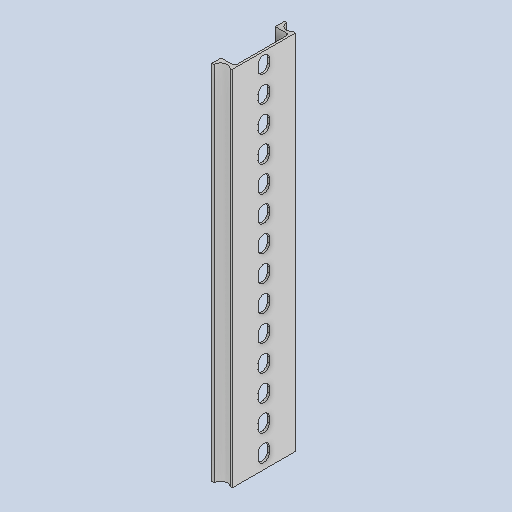
# Autodesk Inventor part: CB_dinrail_mk
Saved by Autodesk Inventor 2022 (Build 260153070, 153G)
## iProperties
Created: 2022-06-25
Part Number: CB_dinrail_mk
Material: アルミニウム 6061-AHC
Document SubType Name: Modeling
Designer: sky
Density: 2.7 g/cm^3
Appearance: アルミニウム - ダーク
Author: sky
Autodesk Inventor part; units mm, degrees
ref_plane "YZ Plane" through (0, 0, 0) normal (1, 0, 0) x (0, 1, 0)
ref_plane "XZ Plane" through (0, 0, 0) normal (0, 1, 0) x (-1, 0, 0)
ref_plane "XY Plane" through (0, 0, 0) normal (0, 0, 1) x (1, 0, 0)
sketch "スケッチ1" plane through (0, 0, 0) normal (0, 1, 0) x (-1, 0, 0)
  line L0 (0, 0) -> (0, -30.5)
  line L1 (7.5, 2.25) -> (7.5, -32.75)
  line L2 (11.9991, -15.25) -> (-11.598, -15.25)
  line L3 (7.5, 2.25) -> (6.5, 2.25)
  line L4 (7.5, 2.25) -> (8.5, 2.25) construction
  line L5 (0, 0) -> (1, 0)
  arc A0 (1, 0) -> (6.5, 2.25) centre (3.2952, 2.2367) ccw
  line L6 (7.5, -32.75) -> (6.5, -32.75)
  line L7 (0, -30.5) -> (1, -30.5)
  arc A1 (6.5, -32.75) -> (1, -30.5) centre (3.2952, -32.7367) ccw
  line L8 (7.5, -2.15) -> (1, -2.15)
  line L9 (1, -2.15) -> (1, -28.35)
  line L10 (1, -28.35) -> (7.5, -28.35)
  dimension "d0" = 30.5
  dimension "d1" = 35
  dimension "d2" = 7.5
  dimension "d3" = 2.25
  dimension "d4" = 1
  dimension "d5" = 180
  dimension "d6" = 1
  dimension "d7" = 4.4
  dimension "d8" = 4.4
  constraints: 22 end point, 5 horizontal, 4 point on circle, 3 symmetric about line, 2 centre point, 2 point on line, 2 vertical, 1 collinear, 1 parallel, 1 perpendicular, 1 other
  measures "d0" distance of L0.start L0.end
  measures "d1" distance of L1.start L1.end
  measures "d2" distance between parallel lines of L1 L0
  measures "d3" vertical distance of L0.start L1.start
  measures "d4" distance of L1.start L3.end
  measures "d5" angle of L3 L4
  measures "d6" distance of L0.start L5.end
  measures "d7" distance between parallel lines of L8 L3
  measures "d8" distance between parallel lines of L10 L6
extrude "押し出し1" add sketch "スケッチ1" along normal blind 175 contours L5 A0 L3 L1 L8 L9 L2 L0 | L2 L9 L10 L1 L6 A1 L7 L0
sketch "スケッチ2" plane through (-1, 0, -28.35) normal (-1, 0, 0) x (0, 0, 1)
  line L0 (0, 0) -> (26.2, 0) projected
  line L1 (26.2, 0) -> (26.2, 175) projected
  line L2 (0, 175) -> (26.2, 175) projected
  line L3 (0, 0) -> (0, 175) projected
  line L4 (15.85, 3) -> (10.35, 3)
  line L5 (10.35, 3) -> (10.35, 11)
  line L6 (10.35, 11) -> (15.85, 11)
  line L7 (15.85, 11) -> (15.85, 3)
  arc A0 (13.1, 3) -> (15.85, 5.75) centre (13.1, 5.75) ccw
  arc A1 (10.35, 5.75) -> (13.1, 3) centre (13.1, 5.75) ccw
  arc A2 (13.1, 11) -> (10.35, 8.25) centre (13.1, 8.25) ccw
  arc A3 (15.85, 8.25) -> (13.1, 11) centre (13.1, 8.25) ccw
  line L8 (15.85, 15.5) -> (10.35, 15.5)
  arc A4 (13.1, 15.5) -> (15.85, 18.25) centre (13.1, 18.25) ccw
  arc A5 (10.35, 18.25) -> (13.1, 15.5) centre (13.1, 18.25) ccw
  arc A6 (15.85, 20.75) -> (13.1, 23.5) centre (13.1, 20.75) ccw
  arc A7 (13.1, 23.5) -> (10.35, 20.75) centre (13.1, 20.75) ccw
  line L9 (10.35, 15.5) -> (10.35, 23.5)
  line L10 (15.85, 23.5) -> (15.85, 15.5)
  line L11 (15.85, 28) -> (10.35, 28)
  arc A8 (13.1, 28) -> (15.85, 30.75) centre (13.1, 30.75) ccw
  arc A9 (10.35, 30.75) -> (13.1, 28) centre (13.1, 30.75) ccw
  arc A10 (15.85, 33.25) -> (13.1, 36) centre (13.1, 33.25) ccw
  arc A11 (13.1, 36) -> (10.35, 33.25) centre (13.1, 33.25) ccw
  line L12 (10.35, 28) -> (10.35, 36)
  line L13 (15.85, 36) -> (15.85, 28)
  line L14 (15.85, 40.5) -> (10.35, 40.5)
  arc A12 (13.1, 40.5) -> (15.85, 43.25) centre (13.1, 43.25) ccw
  arc A13 (10.35, 43.25) -> (13.1, 40.5) centre (13.1, 43.25) ccw
  arc A14 (15.85, 45.75) -> (13.1, 48.5) centre (13.1, 45.75) ccw
  arc A15 (13.1, 48.5) -> (10.35, 45.75) centre (13.1, 45.75) ccw
  line L15 (10.35, 40.5) -> (10.35, 48.5)
  line L16 (15.85, 48.5) -> (15.85, 40.5)
  line L17 (15.85, 53) -> (10.35, 53)
  arc A16 (13.1, 53) -> (15.85, 55.75) centre (13.1, 55.75) ccw
  arc A17 (10.35, 55.75) -> (13.1, 53) centre (13.1, 55.75) ccw
  arc A18 (15.85, 58.25) -> (13.1, 61) centre (13.1, 58.25) ccw
  arc A19 (13.1, 61) -> (10.35, 58.25) centre (13.1, 58.25) ccw
  line L18 (10.35, 53) -> (10.35, 61)
  line L19 (15.85, 61) -> (15.85, 53)
  line L20 (15.85, 65.5) -> (10.35, 65.5)
  arc A20 (13.1, 65.5) -> (15.85, 68.25) centre (13.1, 68.25) ccw
  arc A21 (10.35, 68.25) -> (13.1, 65.5) centre (13.1, 68.25) ccw
  arc A22 (15.85, 70.75) -> (13.1, 73.5) centre (13.1, 70.75) ccw
  arc A23 (13.1, 73.5) -> (10.35, 70.75) centre (13.1, 70.75) ccw
  line L21 (10.35, 65.5) -> (10.35, 73.5)
  line L22 (15.85, 73.5) -> (15.85, 65.5)
  line L23 (15.85, 78) -> (10.35, 78)
  arc A24 (13.1, 78) -> (15.85, 80.75) centre (13.1, 80.75) ccw
  arc A25 (10.35, 80.75) -> (13.1, 78) centre (13.1, 80.75) ccw
  arc A26 (15.85, 83.25) -> (13.1, 86) centre (13.1, 83.25) ccw
  arc A27 (13.1, 86) -> (10.35, 83.25) centre (13.1, 83.25) ccw
  line L24 (10.35, 78) -> (10.35, 86)
  line L25 (15.85, 86) -> (15.85, 78)
  line L26 (15.85, 90.5) -> (10.35, 90.5)
  arc A28 (13.1, 90.5) -> (15.85, 93.25) centre (13.1, 93.25) ccw
  arc A29 (10.35, 93.25) -> (13.1, 90.5) centre (13.1, 93.25) ccw
  arc A30 (15.85, 95.75) -> (13.1, 98.5) centre (13.1, 95.75) ccw
  arc A31 (13.1, 98.5) -> (10.35, 95.75) centre (13.1, 95.75) ccw
  line L27 (10.35, 90.5) -> (10.35, 98.5)
  line L28 (15.85, 98.5) -> (15.85, 90.5)
  line L29 (15.85, 103) -> (10.35, 103)
  arc A32 (13.1, 103) -> (15.85, 105.75) centre (13.1, 105.75) ccw
  arc A33 (10.35, 105.75) -> (13.1, 103) centre (13.1, 105.75) ccw
  arc A34 (15.85, 108.25) -> (13.1, 111) centre (13.1, 108.25) ccw
  arc A35 (13.1, 111) -> (10.35, 108.25) centre (13.1, 108.25) ccw
  line L30 (10.35, 103) -> (10.35, 111)
  line L31 (15.85, 111) -> (15.85, 103)
  line L32 (15.85, 115.5) -> (10.35, 115.5)
  arc A36 (13.1, 115.5) -> (15.85, 118.25) centre (13.1, 118.25) ccw
  arc A37 (10.35, 118.25) -> (13.1, 115.5) centre (13.1, 118.25) ccw
  arc A38 (15.85, 120.75) -> (13.1, 123.5) centre (13.1, 120.75) ccw
  arc A39 (13.1, 123.5) -> (10.35, 120.75) centre (13.1, 120.75) ccw
  line L33 (10.35, 115.5) -> (10.35, 123.5)
  line L34 (15.85, 123.5) -> (15.85, 115.5)
  line L35 (15.85, 128) -> (10.35, 128)
  arc A40 (13.1, 128) -> (15.85, 130.75) centre (13.1, 130.75) ccw
  arc A41 (10.35, 130.75) -> (13.1, 128) centre (13.1, 130.75) ccw
  arc A42 (15.85, 133.25) -> (13.1, 136) centre (13.1, 133.25) ccw
  arc A43 (13.1, 136) -> (10.35, 133.25) centre (13.1, 133.25) ccw
  line L36 (10.35, 128) -> (10.35, 136)
  line L37 (15.85, 136) -> (15.85, 128)
  line L38 (15.85, 140.5) -> (10.35, 140.5)
  arc A44 (13.1, 140.5) -> (15.85, 143.25) centre (13.1, 143.25) ccw
  arc A45 (10.35, 143.25) -> (13.1, 140.5) centre (13.1, 143.25) ccw
  arc A46 (15.85, 145.75) -> (13.1, 148.5) centre (13.1, 145.75) ccw
  arc A47 (13.1, 148.5) -> (10.35, 145.75) centre (13.1, 145.75) ccw
  line L39 (10.35, 140.5) -> (10.35, 148.5)
  line L40 (15.85, 148.5) -> (15.85, 140.5)
  line L41 (15.85, 153) -> (10.35, 153)
  arc A48 (13.1, 153) -> (15.85, 155.75) centre (13.1, 155.75) ccw
  arc A49 (10.35, 155.75) -> (13.1, 153) centre (13.1, 155.75) ccw
  arc A50 (15.85, 158.25) -> (13.1, 161) centre (13.1, 158.25) ccw
  arc A51 (13.1, 161) -> (10.35, 158.25) centre (13.1, 158.25) ccw
  line L42 (10.35, 153) -> (10.35, 161)
  line L43 (15.85, 161) -> (15.85, 153)
  line L44 (15.85, 165.5) -> (10.35, 165.5)
  arc A52 (13.1, 165.5) -> (15.85, 168.25) centre (13.1, 168.25) ccw
  arc A53 (10.35, 168.25) -> (13.1, 165.5) centre (13.1, 168.25) ccw
  arc A54 (15.85, 170.75) -> (13.1, 173.5) centre (13.1, 170.75) ccw
  arc A55 (13.1, 173.5) -> (10.35, 170.75) centre (13.1, 170.75) ccw
  line L45 (10.35, 165.5) -> (10.35, 173.5)
  line L46 (15.85, 173.5) -> (15.85, 165.5)
  line L47 (15.85, 178) -> (10.35, 178)
  arc A56 (13.1, 178) -> (15.85, 180.75) centre (13.1, 180.75) ccw
  arc A57 (10.35, 180.75) -> (13.1, 178) centre (13.1, 180.75) ccw
  arc A58 (15.85, 183.25) -> (13.1, 186) centre (13.1, 183.25) ccw
  arc A59 (13.1, 186) -> (10.35, 183.25) centre (13.1, 183.25) ccw
  line L48 (10.35, 178) -> (10.35, 186)
  line L49 (15.85, 186) -> (15.85, 178)
  line L50 (15.85, 190.5) -> (10.35, 190.5)
  arc A60 (13.1, 190.5) -> (15.85, 193.25) centre (13.1, 193.25) ccw
  arc A61 (10.35, 193.25) -> (13.1, 190.5) centre (13.1, 193.25) ccw
  arc A62 (15.85, 195.75) -> (13.1, 198.5) centre (13.1, 195.75) ccw
  arc A63 (13.1, 198.5) -> (10.35, 195.75) centre (13.1, 195.75) ccw
  line L51 (10.35, 190.5) -> (10.35, 198.5)
  line L52 (15.85, 198.5) -> (15.85, 190.5)
  line L53 (15.85, 203) -> (10.35, 203)
  arc A64 (13.1, 203) -> (15.85, 205.75) centre (13.1, 205.75) ccw
  arc A65 (10.35, 205.75) -> (13.1, 203) centre (13.1, 205.75) ccw
  arc A66 (15.85, 208.25) -> (13.1, 211) centre (13.1, 208.25) ccw
  arc A67 (13.1, 211) -> (10.35, 208.25) centre (13.1, 208.25) ccw
  line L54 (10.35, 203) -> (10.35, 211)
  line L55 (15.85, 211) -> (15.85, 203)
  line L56 (15.85, 215.5) -> (10.35, 215.5)
  arc A68 (13.1, 215.5) -> (15.85, 218.25) centre (13.1, 218.25) ccw
  arc A69 (10.35, 218.25) -> (13.1, 215.5) centre (13.1, 218.25) ccw
  arc A70 (15.85, 220.75) -> (13.1, 223.5) centre (13.1, 220.75) ccw
  arc A71 (13.1, 223.5) -> (10.35, 220.75) centre (13.1, 220.75) ccw
  line L57 (10.35, 215.5) -> (10.35, 223.5)
  line L58 (15.85, 223.5) -> (15.85, 215.5)
  line L59 (15.85, 228) -> (10.35, 228)
  arc A72 (13.1, 228) -> (15.85, 230.75) centre (13.1, 230.75) ccw
  arc A73 (10.35, 230.75) -> (13.1, 228) centre (13.1, 230.75) ccw
  arc A74 (15.85, 233.25) -> (13.1, 236) centre (13.1, 233.25) ccw
  arc A75 (13.1, 236) -> (10.35, 233.25) centre (13.1, 233.25) ccw
  line L60 (10.35, 228) -> (10.35, 236)
  line L61 (15.85, 236) -> (15.85, 228)
  line L62 (15.85, 240.5) -> (10.35, 240.5)
  arc A76 (13.1, 240.5) -> (15.85, 243.25) centre (13.1, 243.25) ccw
  arc A77 (10.35, 243.25) -> (13.1, 240.5) centre (13.1, 243.25) ccw
  arc A78 (15.85, 245.75) -> (13.1, 248.5) centre (13.1, 245.75) ccw
  arc A79 (13.1, 248.5) -> (10.35, 245.75) centre (13.1, 245.75) ccw
  line L63 (10.35, 240.5) -> (10.35, 248.5)
  line L64 (15.85, 248.5) -> (15.85, 240.5)
  line L65 (15.85, 253) -> (10.35, 253)
  arc A80 (13.1, 253) -> (15.85, 255.75) centre (13.1, 255.75) ccw
  arc A81 (10.35, 255.75) -> (13.1, 253) centre (13.1, 255.75) ccw
  arc A82 (15.85, 258.25) -> (13.1, 261) centre (13.1, 258.25) ccw
  arc A83 (13.1, 261) -> (10.35, 258.25) centre (13.1, 258.25) ccw
  line L66 (10.35, 253) -> (10.35, 261)
  line L67 (15.85, 261) -> (15.85, 253)
  line L68 (15.85, 265.5) -> (10.35, 265.5)
  arc A84 (13.1, 265.5) -> (15.85, 268.25) centre (13.1, 268.25) ccw
  arc A85 (10.35, 268.25) -> (13.1, 265.5) centre (13.1, 268.25) ccw
  arc A86 (15.85, 270.75) -> (13.1, 273.5) centre (13.1, 270.75) ccw
  arc A87 (13.1, 273.5) -> (10.35, 270.75) centre (13.1, 270.75) ccw
  line L69 (10.35, 265.5) -> (10.35, 273.5)
  line L70 (15.85, 273.5) -> (15.85, 265.5)
  line L71 (15.85, 278) -> (10.35, 278)
  arc A88 (13.1, 278) -> (15.85, 280.75) centre (13.1, 280.75) ccw
  arc A89 (10.35, 280.75) -> (13.1, 278) centre (13.1, 280.75) ccw
  arc A90 (15.85, 283.25) -> (13.1, 286) centre (13.1, 283.25) ccw
  arc A91 (13.1, 286) -> (10.35, 283.25) centre (13.1, 283.25) ccw
  line L72 (10.35, 278) -> (10.35, 286)
  line L73 (15.85, 286) -> (15.85, 278)
  line L74 (15.85, 290.5) -> (10.35, 290.5)
  arc A92 (13.1, 290.5) -> (15.85, 293.25) centre (13.1, 293.25) ccw
  arc A93 (10.35, 293.25) -> (13.1, 290.5) centre (13.1, 293.25) ccw
  arc A94 (15.85, 295.75) -> (13.1, 298.5) centre (13.1, 295.75) ccw
  arc A95 (13.1, 298.5) -> (10.35, 295.75) centre (13.1, 295.75) ccw
  line L75 (10.35, 290.5) -> (10.35, 298.5)
  line L76 (15.85, 298.5) -> (15.85, 290.5)
  line L77 (15.85, 303) -> (10.35, 303)
  arc A96 (13.1, 303) -> (15.85, 305.75) centre (13.1, 305.75) ccw
  arc A97 (10.35, 305.75) -> (13.1, 303) centre (13.1, 305.75) ccw
  arc A98 (15.85, 308.25) -> (13.1, 311) centre (13.1, 308.25) ccw
  arc A99 (13.1, 311) -> (10.35, 308.25) centre (13.1, 308.25) ccw
  line L78 (10.35, 303) -> (10.35, 311)
  line L79 (15.85, 311) -> (15.85, 303)
  point P0 (28.35, 0)
  dimension "d11" = 5.5
  dimension "d12" = 8
  dimension "d13" = 10.35
  dimension "d14" = 3
  dimension "d16" = 2.75
  dimension "d18" = 2.75
  dimension "d21" = 12.5
  constraints: 200 point on circle, 152 end point, 100 centre point, 100 point on line, 26 midpoint, 2 parallel, 1 collinear, 1 horizontal, 1 perpendicular, 1 vertical, 455 other
  measures "d11" distance of L5.end L6.end
  measures "d12" distance of L4.end L5.end
  measures "d13" distance between parallel lines of L3 L5
  measures "d14" distance between parallel lines of L0 L4
  measures "d16" distance from line of L6 A2.centre
  measures "d18" distance from line of L4 A0.centre
  measures "d21" distance of L4.start L8.start
extrude "押し出し2" cut sketch "スケッチ2" against normal blind 3 contours A1 L5 A2 A3 L7 A0 | A5 L9 A7 A6 L10 A4 | A9 L12 A11 A10 L13 A8 | A13 L15 A15 A14 L16 A12 | A17 L18 A19 A18 L19 A16 | A21 L21 A23 A22 L22 A20 | A25 L24 A27 A26 L25 A24 | A29 L27 A31 A30 L28 A28 | A33 L30 A35 A34 L31 A32 | A37 L33 A39 A38 L34 A36 | A41 L36 A43 A42 L37 A40 | A45 L39 A47 A46 L40 A44 | A49 L42 A51 A50 L43 A48 | A53 L45 A55 A54 L46 A52 | A57 L48 A59 A58 L49 A56 | A61 L51 A63 A62 L52 A60 | A65 L54 A67 A66 L55 A64 | A69 L57 A71 A70 L58 A68 | A73 L60 A75 A74 L61 A72 | A77 L63 A79 A78 L64 A76 | A81 L66 A83 A82 L67 A80 | A85 L69 A87 A86 L70 A84 | A89 L72 A91 A90 L73 A88 | A93 L75 A95 A94 L76 A92
fillet "フィレット1" radius 1 2 edges at (-1, 87.5, -28.35) (-1, 87.5, -2.15)
